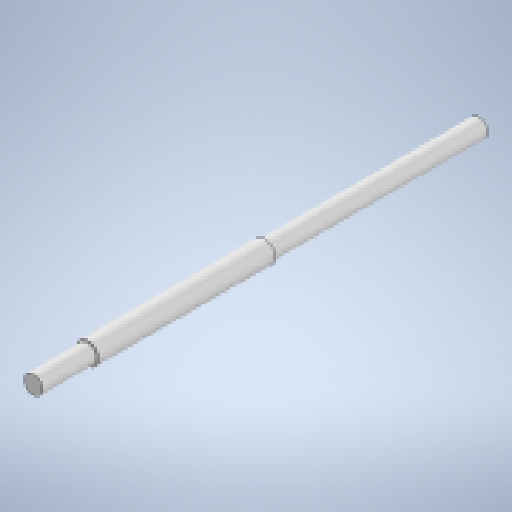
# Autodesk Inventor part: os_napedowa
Saved by Autodesk Inventor 2023 (Build 270158000, 158)
## iProperties
Created: 2023-01-19
Part Number: os_napedowa
Material: Generic
Document SubType Name: Modeling
Designer: komputer
Density: 1 g/cm^3
Appearance: Default
Mass: 16.4305 g
Surface Area: 68.8009 cm^2
Volume: 16.4305 cm^3
Author: komputer
Autodesk Inventor part; units mm, degrees
ref_plane "YZ Plane" through (0, 0, 0) normal (1, 0, 0) x (0, 1, 0)
sketch "Sketch1" plane through (0, 0, 0) normal (0, 0, 1) x (1, 0, 0)
  circle A0 centre (0, 0) radius 7.5 projected
  circle A1 centre (0, 0) radius 5.5 projected
  circle A2 centre (0, 0) radius 5 projected
extrude "Extrusion1" add sketch "Sketch1" against normal blind 50 contours A2
sketch "Sketch2" plane through (0, 0, 0) normal (0, 0, 1) x (1, 0, 0)
  point P0 (0, 0)
sketch "Sketch3" plane through (0, 0, 0) normal (0, 0, 1) x (1, 0, 0)
  circle A0 centre (0, 0) radius 5 projected
extrude "Extrusion2" add sketch "Sketch3" along normal blind 150
sketch "Sketch4" plane through (0, 0, 150) normal (0, 0, 1) x (1, 0, 0)
  circle A0 centre (0, 0) radius 5 projected
  circle A1 centre (0, 0) radius 4
  dimension "d4" = 8
  constraints: 1 centre point, 1 coincident
  measures "d4" diameter of A1
extrude "Extrusion3" cut sketch "Sketch4" against normal blind 30
sketch "Sketch5" plane through (0, 0, -50) normal (0, 0, -1) x (-1, 0, 0)
  circle A0 centre (0, 0) radius 5 projected
extrude "Extrusion4" add sketch "Sketch5" along normal blind 20
sketch "Szkic6" plane through (0, 0, -70) normal (0, 0, -1) x (-1, 0, 0)
  circle A0 centre (0, 0) radius 4 projected
  circle A1 centre (0, 0) radius 5
  constraints: 1 centre point, 2 other
extrude "Wyciągnięcie proste5" add sketch "Szkic6" along normal blind 6 contours A0 | A1
sketch "Szkic7" plane through (0, 0, 150) normal (0, 0, 1) x (1, 0, 0)
  circle A0 centre (0, 0) radius 5 projected
  circle A1 centre (0, 0) radius 5 projected
ref_plane "Płaszczyzna konstrukcyjna1" through (-9.4999, -9.4999, 27.64) normal (0, 0, 1) x (0.8774, -0.4797, 0)
extrude "Wyciągnięcie proste6" cut sketch "Szkic7" against normal up to surface (122.36 mm away)
sketch "Szkic8" plane through (0, 0, 27.64) normal (0, 0, 1) x (1, 0, 0)
  circle A0 centre (0, 0) radius 5 projected
  circle A1 centre (0, 0) radius 4.4644
  point P0 (0, 0)
  constraints: 1 centre point, 1 coincident
extrude "Wyciągnięcie proste7" add sketch "Szkic8" along normal blind 2 contours A1
sketch "Szkic9" plane through (0, 0, 29.64) normal (0, 0, 1) x (1, 0, 0)
  circle A0 centre (0, 0) radius 4.4644 projected
  circle A1 centre (0, 0) radius 5 projected
  point P0 (0, 0)
ref_plane "Płaszczyzna konstrukcyjna2" through (-6.6123, -6.6123, 155) normal (0, 0, -1) x (-0.1077, 0.9942, 0)
extrude "Wyciągnięcie proste8" add sketch "Szkic9" along normal up to surface (125.36 mm away) contours A0 | A1
sketch "Szkic10" plane through (0, 0, -76) normal (0, 0, -1) x (-1, 0, 0)
  circle A0 centre (0, 0) radius 5 projected
  point P0 (0, 0)
extrude "Wyciągnięcie proste9" add sketch "Szkic10" along normal blind 15
sketch "Szkic11" plane through (0, 0, 27.64) normal (0, 0, 1) x (1, 0, 0)
  circle A0 centre (0, 0) radius 5 projected
  circle A1 centre (0, 0) radius 4.4644 projected
  circle A2 centre (0, 0) radius 6
  point P0 (0, 0)
  dimension "d19" = 12
  constraints: 1 centre point, 1 coincident
  measures "d19" diameter of A2
extrude "Wyciągnięcie proste10" add sketch "Szkic11" along normal blind 97.36 contours A0 | A1 | A2
sketch "Szkic12" plane through (0, 0, -91) normal (0, 0, -1) x (-1, 0, 0)
  circle A0 centre (0, 0) radius 5 projected
  point P0 (0, 0)
extrude "Wyciągnięcie proste11" cut sketch "Szkic12" against normal blind 0.6
sketch "Szkic13" plane through (0, 0, -90.4) normal (0, 0, -1) x (-1, 0, 0)
  circle A0 centre (0, 0) radius 5 projected
extrude "Wyciągnięcie proste12" cut sketch "Szkic13" against normal blind 0.04
sketch "Szkic14" plane through (0, 0, 125) normal (0, 0, 1) x (1, 0, 0)
  circle A0 centre (0, 0) radius 6 projected
  circle A1 centre (0, 0) radius 5 projected
  point P0 (0, 0)
extrude "Wyciągnięcie proste13" cut sketch "Szkic14" against normal blind 0.36
sketch "Szkic15" plane through (0, 0, 155) normal (0, 0, 1) x (1, 0, 0)
  circle A0 centre (0, 0) radius 5 projected
  point P0 (0, 0)
extrude "Wyciągnięcie proste14" cut sketch "Szkic15" against normal blind 0.36
body "Solid1"
